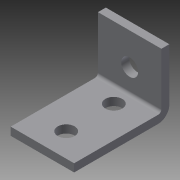
# Autodesk Inventor part: Gusset 5
Saved by Autodesk Inventor 2013 (Build 170138000, 138)
## iProperties
Created: 2013-01-31
Part Number: Gusset 5
Material: Generic
Document SubType Name: Sheet Metal
Designer: actoennies
Density: 1 g/cm^3
Sheet Metal Rule: Default
Author: actoennies
Autodesk Inventor part; units mm, degrees
ref_plane "YZ Plane" through (0, 0, 0) normal (1, 0, 0) x (0, 1, 0)
ref_plane "XZ Plane" through (0, 0, 0) normal (0, 1, 0) x (-1, 0, 0)
ref_plane "XY Plane" through (0, 0, 0) normal (0, 0, 1) x (1, 0, 0)
sketch "Sketch1" plane through (0, 0, 0) normal (0, 1, 0) x (-1, 0, 0)
  line L0 (0, 0) -> (25.4, 0)
  line L1 (25.4, 0) -> (25.4, 38.1)
  line L2 (25.4, 38.1) -> (0, 38.1)
  line L3 (0, 38.1) -> (0, 0)
  circle A0 centre (12.7, 9.525) radius 3.3782
  circle A1 centre (12.7, 28.575) radius 3.3782
  dimension "d0" = 25.4
  dimension "d1" = 38.1
  dimension "d2" = 6.7564
  dimension "d3" = 6.7564
  dimension "d4" = 9.525
  dimension "d5" = 9.525
  dimension "d6" = 12.7
  dimension "d7" = 12.7
  measures "d0" distance of L0.start L0.end
  measures "d1" distance of L0.end L1.end
  measures "d2" diameter of A0
  measures "d3" diameter of A1
  measures "d4" distance from line of L2 A1.centre
  measures "d5" distance from line of L0 A0.centre
  measures "d6" distance from line of L1 A0.centre
  measures "d7" distance from line of L1 A1.centre
extrude "Plate1" add sketch "Sketch1" along normal blind 3.175
sketch "Sketch2" plane through (-25.4, 0, 3.175) normal (0, 0, -1) x (-1, 0, 0)
  line L0 (-25.4, 0) -> (0, 0)
  line L1 (0, 0) -> (0, 25.4)
  line L2 (0, 25.4) -> (-25.4, 25.4)
  line L3 (-25.4, 25.4) -> (-25.4, 0)
  constraints: 6 end point, 1 horizontal, 1 perpendicular, 1 vertical
edge flange "Flange1" height 25.4 angle 90 thickness 3.175 bend radius 1.27 thickness toward (0, 0, -1) relief straight relief width 3.175 relief depth 1.5875 edges at (-12.7, 3.175, 0) wall of the first edge with corners at (0, 0, 3.175) (-25.4, 0, 3.175) (-25.4, 25.4, 3.175) (0, 25.4, 3.175)
bend "Bend1"
corner "Corner1"
sketch "Sketch3" plane through (-25.4, 25.4, 3.175) normal (0, 0, 1) x (1, 0, 0)
  line L0 (25.4, 0) -> (0, 0) projected
  line L1 (0, 0) -> (0, -20.955) projected
  circle A0 centre (12.7, -12.7) radius 3.3782
  point P0 (25.4, -25.4)
  dimension "d19" = 6.7564
  dimension "d20" = 12.7
  dimension "d21" = 12.7
  constraints: 1 centre point
  measures "d19" diameter of A0
  measures "d20" distance from line of L0 A0.centre
  measures "d21" distance from line of L1 A0.centre
extrude "Cut1" cut sketch "Sketch3" against normal blind 3.175
equation "\"d22\" = Thickness"
equation "\"d9\" = BendReliefWidth"
equation "\"d10\" = BendReliefDepth"
equation "\"d11\" = MinimumRemnant"
equation "\"d12\" = BendRadius"
equation "\"d16\" = CornerReliefSize"
equation "\"d17\" = GapSize"
equation "\"d18\" = JacobiRadiusSize"
equation "\"BendRadius\" = Thickness"
equation "\"BendReliefWidth\" = Thickness"
equation "\"BendReliefDepth\" = 0.5 * Thickness"
equation "\"CornerReliefSize\" = 4 * Thickness"
equation "\"MinimumRemnant\" = 2 * Thickness"
equation "\"TransitionRadius\" = BendRadius"
equation "\"JacobiRadiusSize\" = BendRadius"
equation "\"GapSize\" = Thickness"
equation "\"d8\" = BendRadius"
equation "\"Thickness\" = 3.175"
body "Solid1"
